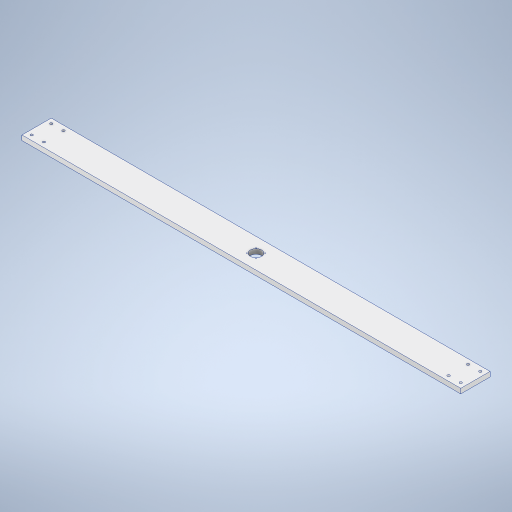
# Autodesk Inventor part: Traversa_chiusura
Saved by Autodesk Inventor 2024.2 (Build 282272000, 272)
## iProperties
Created: 2024-03-18
Part Number: Traversa_chiusura
Material: Aluminum 6061
Document SubType Name: Modeling
Designer: feder
Density: 2.7 g/cm^3
Appearance: Aluminum - Flat
Author: feder
Autodesk Inventor part; units mm, degrees
ref_plane "YZ Plane" through (0, 0, 0) normal (1, 0, 0) x (0, 1, 0)
ref_plane "XZ Plane" through (0, 0, 0) normal (0, 1, 0) x (-1, 0, 0)
ref_plane "XY Plane" through (0, 0, 0) normal (0, 0, 1) x (1, 0, 0)
sketch "Sketch1" plane through (0, 0, 0) normal (0, 1, 0) x (-1, 0, 0)
  line L0 (-4500, 300) -> (-4500, -300)
  line L1 (4050, -300) -> (4500, -300)
  line L2 (-4500, 300) -> (4500, 300)
  line L3 (4500, 300) -> (4500, -300)
  line L4 (4500, -300) -> (-4500, -300)
  line L5 (-4500, -300) -> (-4500, 300)
  line L6 (4050, -300) -> (4500, -300)
  line L7 (4500, -300) -> (4500, 300)
  line L8 (4500, 300) -> (4050, 300)
  line L9 (4050, 300) -> (4050, -300) construction
  line L10 (4150, -300) -> (4150, 200) construction
  line L11 (4150, 200) -> (4500, 200) construction
  line L12 (4050, -200) -> (4500, -200) construction
  line L13 (4400, 300) -> (4400, -300) construction
  circle A0 centre (4400, -200) radius 25
  circle A1 centre (4150, -200) radius 25
  circle A2 centre (4400, 200) radius 25
  circle A3 centre (4150, 200) radius 25
  line L14 (0, -4359.7142) -> (0, 4067.2599) construction
  line L15 (-4050, -300) -> (-4500, -300)
  line L16 (-4500, 300) -> (-4500, -300)
  line L17 (-4050, -300) -> (-4500, -300)
  line L18 (-4500, -300) -> (-4500, 300)
  line L19 (-4500, 300) -> (-4050, 300)
  line L20 (-4050, 300) -> (-4050, -300) construction
  line L21 (-4150, -300) -> (-4150, 200) construction
  line L22 (-4150, 200) -> (-4500, 200) construction
  line L23 (-4050, -200) -> (-4500, -200) construction
  line L24 (-4400, 300) -> (-4400, -300) construction
  circle A4 centre (-4400, -200) radius 25
  circle A5 centre (-4150, -200) radius 25
  circle A6 centre (-4400, 200) radius 25
  circle A7 centre (-4150, 200) radius 25
  circle A8 centre (0, 0) radius 132.5
  line L25 (0, 0) -> (90.1995, 90.1995) construction
  line L26 (0, 0) -> (127.5614, 0) construction
  line L27 (93.6915, 93.6915) -> (-93.6915, 93.6915)
  line L28 (-93.6915, 93.6915) -> (-93.6915, -93.6915)
  line L29 (-93.6915, -93.6915) -> (93.6915, -93.6915)
  line L30 (93.6915, -93.6915) -> (93.6915, 93.6915)
  line L31 (93.6915, 93.6915) -> (-93.6915, -93.6915) construction
  line L32 (-93.6915, 93.6915) -> (93.6915, -93.6915) construction
  line L33 (93.6915, -93.6915) -> (0, 0)
  circle A9 centre (93.6915, -93.6915) radius 7.5
  circle A10 centre (-93.6915, -93.6915) radius 7.5
  circle A11 centre (93.6915, 93.6915) radius 7.5
  circle A12 centre (-93.6915, 93.6915) radius 7.5
  circle A13 centre (0, 0) radius 115
  dimension "d0" = 9000
  dimension "d1" = 600
  dimension "d2" = 300
  dimension "d5" = 450
  dimension "d6" = 100
  dimension "d7" = 100
  dimension "d8" = 100
  dimension "d9" = 50
  dimension "d10" = 50
  dimension "d11" = 50
  dimension "d12" = 50
  dimension "d13" = 265
  dimension "d16" = 45
  dimension "d22" = 187.383
  dimension "d23" = 187.383
  dimension "d24" = 15
  dimension "d25" = 15
  dimension "d26" = 15
  dimension "d27" = 15
  dimension "d28" = 230
  constraints: 68 end point, 15 symmetric about line, 14 centre point, 12 point on line, 9 coincident, 8 parallel, 4 horizontal, 3 perpendicular, 2 midpoint, 1 collinear, 1 equal length, 1 vertical, 5 other
  measures "d0" distance between parallel lines of L0 L3
  measures "d1" distance between parallel lines of L2 L4
  measures "d2" distance from line of point (0, 0) L4
  measures "d5" distance between parallel lines of L3 L9
  measures "d6" distance between parallel lines of L9 L10
  measures "d7" distance between parallel lines of L1 L12
  measures "d8" distance between parallel lines of L3 L13
  measures "d9" diameter of A0
  measures "d10" diameter of A1
  measures "d11" diameter of A2
  measures "d12" diameter of A3
  measures "d13" diameter of A8
  measures "d16" angle of L26 L25
  measures "d22" distance of L29.end L28.end
  measures "d23" distance of L28.end L27.end
  measures "d24" diameter of A9
  measures "d25" diameter of A10
  measures "d26" diameter of A11
  measures "d27" diameter of A12
  measures "d28" diameter of A13
extrude "Extrusion1" add sketch "Sketch1" along normal blind 100 contours L2 L3 L1 L4 L0 | A8 A9 L30 A13 A11 | L30 A13 L27 A11 | A9 L33 A13 L30 | A11 L27 A13 A12 A8 | A8 A10 L29 A13 A9 | L29 A13 L33 A9 | L27 A13 L28 A12 | A12 L28 A13 A10 A8 | A10 L28 A13 L29
body "Solid1"
